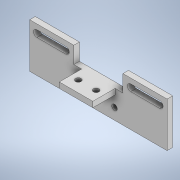
# Autodesk Inventor part: 20230309gamma
Saved by Autodesk Inventor 2020 (Build 240168000, 168)
## iProperties
Created: 2022-08-31
Part Number: 20230309gamma
Material: 一般
Document SubType Name: Modeling
Designer: Naggy
Density: 1 g/cm^3
Appearance: 既定
Author: Naggy
Autodesk Inventor part; units mm, degrees
ref_plane "YZ Plane" through (0, 0, 0) normal (1, 0, 0) x (0, 1, 0)
ref_plane "XZ Plane" through (0, 0, 0) normal (0, 1, 0) x (-1, 0, 0)
ref_plane "XY Plane" through (0, 0, 0) normal (0, 0, 1) x (1, 0, 0)
sketch "スケッチ1" plane through (0, 0, 0) normal (0, 0, 1) x (1, 0, 0)
  line L0 (-61.5, -20) -> (61.5, -20)
  line L1 (61.5, -20) -> (61.5, 20)
  line L2 (61.5, 20) -> (-61.5, 20)
  line L3 (-61.5, 20) -> (-61.5, -20)
  line L4 (-61.5, -20) -> (61.5, 20) construction
  line L5 (61.5, -20) -> (-61.5, 20) construction
  point P0 (0, 0)
  dimension "d0" = 123
  dimension "d1" = 40
  constraints: 12 end point, 2 midpoint, 2 parallel, 1 horizontal, 1 perpendicular
  measures "d0" distance between parallel lines of L1 L3
  measures "d1" distance between parallel lines of L0 L2
extrude "押し出し1" add sketch "スケッチ1" along normal blind 5
sketch "スケッチ2" plane through (0, 0, 5) normal (0, 0, 1) x (1, 0, 0)
  line L0 (61.5, 20) -> (-61.5, 20) projected
  line L1 (0, 20) -> (22, 20)
  line L2 (22, 20) -> (22, 5)
  line L3 (22, 5) -> (0, 5)
  line L4 (0, 5) -> (0, 20)
  line L5 (0, 20) -> (-22, 20)
  line L6 (-22, 20) -> (-22, 5)
  line L7 (-22, 5) -> (0, 5)
  line L8 (0, 5) -> (0, 20)
  point P0 (0, 0)
  dimension "d4" = 22
  dimension "d5" = 15
  dimension "d6" = 22
  constraints: 16 end point, 4 parallel, 2 horizontal, 2 perpendicular, 1 midpoint
  measures "d4" distance between parallel lines of L2 L4
  measures "d5" distance between parallel lines of L3 L0
  measures "d6" distance between parallel lines of L6 L4
extrude "押し出し2" cut sketch "スケッチ2" against normal blind 5
sketch "スケッチ3" plane through (0, 0, 5) normal (0, 0, 1) x (1, 0, 0)
  line L0 (61.5, 20) -> (22, 20) projected
  line L1 (-22, 5) -> (-22, 20) projected
  line L2 (22, 20) -> (22, 5) projected
  line L3 (-29, 12.5) -> (-55, 12.5) construction
  line L4 (-29, 15.5) -> (-55, 15.5)
  line L5 (-55, 9.5) -> (-29, 9.5)
  arc A0 (-29, 9.5) -> (-29, 15.5) centre (-29, 12.5) ccw
  arc A1 (-55, 15.5) -> (-55, 9.5) centre (-55, 12.5) ccw
  line L6 (55, 12.5) -> (29, 12.5) construction
  line L7 (55, 15.5) -> (29, 15.5)
  line L8 (29, 9.5) -> (55, 9.5)
  arc A2 (55, 9.5) -> (55, 15.5) centre (55, 12.5) ccw
  arc A3 (29, 15.5) -> (29, 9.5) centre (29, 12.5) ccw
  point P0 (0, 0)
  point P1 (42, 12.5)
  point P2 (-42, 12.5)
  dimension "d9" = 7.5
  dimension "d10" = 20
  dimension "d11" = 20
  dimension "d12" = 32
  dimension "d13" = 6
  dimension "d14" = 32
  dimension "d15" = 6
  constraints: 16 end point, 8 point on circle, 8 tangent, 4 centre point, 2 horizontal, 2 midpoint, 2 parallel
  measures "d9" distance from line of point (42, 12.5) L0
  measures "d10" distance from line of point (-42, 12.5) L1
  measures "d11" distance from line of point (42, 12.5) L2
  measures "d13" distance between parallel lines of L5 L4
  measures "d15" distance between parallel lines of L8 L7
extrude "押し出し3" cut sketch "スケッチ3" against normal blind 5
sketch "スケッチ4" plane through (0, 0, 5) normal (0, 0, 1) x (1, 0, 0)
  line L0 (-61.5, -20) -> (61.5, -20) projected
  line L1 (61.5, -20) -> (61.5, 20) projected
  line L2 (-61.5, 20) -> (-61.5, -20) projected
  point P0 (0, 0)
  point P1 (14.5, -10)
  point P2 (-14.5, -10)
  dimension "d18" = 10
  dimension "d19" = 47
  dimension "d20" = 47
  dimension "d21" = 10
  measures "d18" distance from line of point (14.5, -10) L0
  measures "d19" distance from line of point (14.5, -10) L1
  measures "d20" distance from line of point (-14.5, -10) L2
  measures "d21" distance from line of L0 point (-14.5, -10)
hole "穴1" at (14.5, -10, 5) at (-14.5, -10, 5) direction (0, 0, -1) diameter 5 depth 8.8 tip angle 118
sketch "スケッチ5" plane through (0, 0, 5) normal (0, 0, 1) x (1, 0, 0)
  line L0 (-22, 5) -> (22, 5) projected
  line L1 (0, 5) -> (-15, 5)
  line L2 (-15, 5) -> (-15, 0)
  line L3 (-15, 0) -> (0, 0)
  line L4 (0, 0) -> (0, 5)
  line L5 (0, 0) -> (15, 0)
  line L6 (15, 0) -> (15, 5)
  line L7 (15, 5) -> (0, 5)
  line L8 (0, 5) -> (0, 0)
  point P0 (0, 0)
  dimension "d29" = 15
  dimension "d30" = 15
  constraints: 16 end point, 4 parallel, 2 horizontal, 2 perpendicular, 1 midpoint, 1 point on line
  measures "d29" distance between parallel lines of L4 L2
  measures "d30" distance between parallel lines of L6 L4
extrude "押し出し4" add sketch "スケッチ5" along normal blind 20
sketch "スケッチ6" plane through (-15, 0, 5) normal (0, -1, 0) x (1, 0, 0)
  point P0 (15, -5)
sketch "スケッチ7" plane through (-22, 5, 0) normal (0, 1, 0) x (1, 0, 0)
  line L0 (37, -25) -> (7, -25) projected
  line L1 (37, -5) -> (37, -25) projected
  line L2 (7, -5) -> (7, -25) projected
  point P0 (22, 0)
  point P1 (30, -15)
  point P2 (14, -15)
  dimension "d33" = 10
  dimension "d34" = 10
  dimension "d35" = 7
  dimension "d36" = 7
  measures "d33" distance from line of point (30, -15) L0
  measures "d34" distance from line of point (14, -15) L0
  measures "d35" distance from line of point (30, -15) L1
  measures "d36" distance from line of L2 point (14, -15)
hole "穴2" at (8, 5, 15) at (-8, 5, 15) direction (0, -1, 0) diameter 5 depth 8.8 tip angle 118
